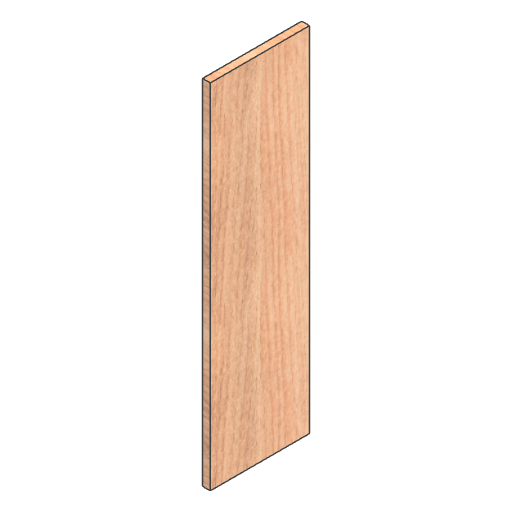
# Autodesk Inventor part: CUT PART C-01
Saved by Autodesk Inventor 2023.2 (Build 272271000, 271)
## iProperties
Created: 2022-11-02
Part Number: CUT PART C-01
Material: Wood (Birch)
Document SubType Name: Modeling
Designer: GUT
Density: 0.55 g/cm^3
Appearance: Birch - Natural Polished
Mass: 550.341 g
Surface Area: 1835.22 cm^2
Volume: 1000.62 cm^3
b: 545,000 mm
d1: 153,000 mm
d2: 12,000 mm
d3: 0,00 deg
Author: GUT
Autodesk Inventor part; units mm, degrees
ref_plane "YZ Plane" through (0, 0, 0) normal (1, 0, 0) x (0, 1, 0)
ref_plane "XZ Plane" through (0, 0, 0) normal (0, 1, 0) x (-1, 0, 0)
ref_plane "XY Plane" through (0, 0, 0) normal (0, 0, 1) x (1, 0, 0)
sketch "Sketch1" plane through (0, 0, 0) normal (1, 0, 0) x (0, 1, 0)
  line L0 (137.431, 17.6667) -> (682.431, 17.6667)
  line L1 (682.431, 17.6667) -> (682.431, -135.3333)
  line L2 (682.431, -135.3333) -> (137.431, -135.3333)
  line L3 (137.431, -135.3333) -> (137.431, 17.6667)
  point P0 (0, 0)
  dimension "b" = 545
  dimension "d1" = 153
  constraints: 8 end point, 2 parallel, 1 horizontal, 1 perpendicular
  measures "b" distance of L1.end L2.end
  measures "d1" distance of L0.end L1.end
extrude "Extrusion1" add sketch "Sketch1" along normal blind 12
body "Solid1"
